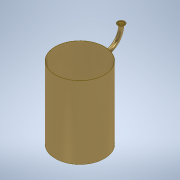
# Autodesk Inventor part: still
Saved by Autodesk Inventor 2020 (Build 240168000, 168)
## iProperties
Created: 2022-08-31
Part Number: still
Material: Gold
Document SubType Name: Modeling
Designer: Intuito_PC
Density: 19.3 g/cm^3
Appearance: Foil Gold
Author: Intuito_PC
Autodesk Inventor part; units mm, degrees
ref_plane "YZ Plane" through (0, 0, 0) normal (1, 0, 0) x (0, 1, 0)
ref_plane "XZ Plane" through (0, 0, 0) normal (0, 1, 0) x (-1, 0, 0)
ref_plane "XY Plane" through (0, 0, 0) normal (0, 0, 1) x (1, 0, 0)
sketch "Sketch1" plane through (0, 0, 0) normal (0, 1, 0) x (-1, 0, 0)
  circle A0 centre (0, 0) radius 295
  dimension "d0" = 590
  constraints: 1 centre point, 1 coincident
  measures "d0" diameter of A0
extrude "Extrusion1" add sketch "Sketch1" along normal blind 870
shell "Shell1" thickness 3 removed faces 1 at (-9.963, 870, -139.7076)
sketch "Sketch2" plane through (0, 0, 0) normal (1, 0, 0) x (0, 1, 0)
  line L0 (990, -495) -> (1010, -495)
  line L1 (870, -295) -> (870, 295) projected
  line L2 (870, -295) -> (670, -295)
  line L3 (0, -295) -> (870, -295) projected
  arc A0 (790, -295) -> (990, -495) centre (990, -295) ccw
  line L4 (3, -292) -> (870, -292) projected
  line L5 (790, -295) -> (840.8, -295)
  line L6 (790.0347, -291.2721) -> (790, -291.2721)
  line L7 (790, -292) -> (790, -291.2721)
  line L8 (790, -295) -> (790, -280.1792)
  point P0 (0, 0)
  point P1 (790, -495)
  dimension "d5" = 200
  dimension "d6" = 200
  dimension "d7" = 220
  dimension "d8" = 200
  dimension "d16" = 50.8
  constraints: 12 end point, 4 point on line, 3 point on circle, 1 centre point, 1 horizontal, 1 perpendicular, 1 tangent, 1 vertical
  measures "d5" distance of L1.start L2.end
  measures "d6" distance between parallel lines of L2 L0
  measures "d7" distance of point (790, -495) L0.end
  measures "d8" radius of A0
  measures "d16" distance of L5.start L5.end
ref_plane "Work Plane1" through (0, 1010, -495) normal (0, 1, 0) x (-1, 0, 0)
sketch "Sketch3" plane through (0, 1010, -495) normal (0, 1, 0) x (-1, 0, 0)
  circle A0 centre (0, 0) radius 25
  point P0 (0, 495)
  dimension "d9" = 50
  constraints: 1 centre point
  measures "d9" diameter of A0
sweep "Sweep1" add profiles "Sketch3" path "Sketch2" path curves L0 A0
sketch "Sketch4" plane through (0, 1010, -495) normal (0, 1, 0) x (1, 0, 0)
  circle A0 centre (0, 0) radius 25 projected
  circle A1 centre (0, 0) radius 24
  point P0 (0, -495)
  dimension "d13" = 48
  constraints: 1 centre point, 1 coincident
  measures "d13" diameter of A1
sweep "Sweep2" cut profiles "Sketch4" path "Sketch2" path curves L0 A0 contours A1
sketch "Sketch5" plane through (0, 1010, -495) normal (0, 1, 0) x (1, 0, 0)
  circle A0 centre (0, 0) radius 42.5
  point P0 (0, -495)
  dimension "d17" = 85
  constraints: 1 centre point
  measures "d17" diameter of A0
extrude "Extrusion2" add sketch "Sketch5" along normal blind 2
sketch "Sketch6" plane through (0, 1010, -495) normal (0, 1, 0) x (-1, 0, 0)
  circle A0 centre (0, 0) radius 24
  point P0 (0, 495)
  dimension "d20" = 48
  constraints: 1 centre point
  measures "d20" diameter of A0
extrude "Extrusion3" cut sketch "Sketch6" against normal mid plane 5
sketch "Sketch7" plane through (0, 1012, -495) normal (0, 1, 0) x (1, 0, 0)
  circle A0 centre (0, 0) radius 42.5 projected
  point P0 (0, -495)
  point P1 (0.0517, 33.6296)
  dimension "d30" = 33.6296
  measures "d30" distance of A0.centre point (0.052, 33.63)
hole "Hole1" at (0.0517, 1012, -528.6296) direction (0, -1, 0) diameter 8 depth 10 tip angle 118
pattern_circular "Circular Pattern1" count 4 over 360 about axis through (0, 1010, -495) along (0, -1, 0) of "Hole1"
fillet "Fillet1" radius 3.175 1 edges at (295, 0, 0)
body "Solid1"
